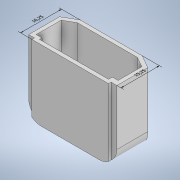
# Autodesk Inventor part: Sarten
Saved by Autodesk Inventor 2020.3 (Build 243373000, 373)
## iProperties
Created: 2021-01-09
Part Number: Sarten
Material: Generic
Document SubType Name: Modeling
Designer: super
Density: 1 g/cm^3
Appearance: Default
Author: super
Autodesk Inventor part; units mm, degrees
ref_plane "YZ Plane" through (0, 0, 0) normal (1, 0, 0) x (0, 1, 0)
ref_plane "XZ Plane" through (0, 0, 0) normal (0, 1, 0) x (-1, 0, 0)
ref_plane "XY Plane" through (0, 0, 0) normal (0, 0, 1) x (1, 0, 0)
sketch "Sketch1" plane through (0, 0, 0) normal (0, 1, 0) x (-1, 0, 0)
  line L0 (0, 0) -> (-35, 0)
  line L1 (-35, 0) -> (-35, -35)
  line L2 (-35, -35) -> (0, -35)
  line L3 (0, -35) -> (0, 0)
  dimension "d0" = 35
  dimension "d1" = 35
  constraints: 8 end point, 2 parallel, 1 horizontal, 1 perpendicular
  measures "d0" distance of L2.end L1.end
  measures "d1" distance of L1.end L0.end
extrude "Extrusion1" add sketch "Sketch1" along normal blind 28
sketch "Sketch2" plane through (0, 28, 0) normal (0, 1, 0) x (1, 0, 0)
  line L0 (35, 19) -> (32.7, 19)
  line L1 (32.7, 19) -> (32.7, 17)
  line L2 (35, 19) -> (35, 17.125)
  line L3 (32.7, 17) -> (35, 17)
  line L4 (35, 17) -> (35, 17.125)
  point P0 (0, 0)
  point P1 (35, 35)
  dimension "d6" = 16
  dimension "d7" = 2.3
  dimension "d8" = 2
  constraints: 10 end point, 2 horizontal, 2 perpendicular
  measures "d6" distance of point (35, 35) L0.start
  measures "d7" distance of L0.start L0.end
  measures "d8" distance of L0.end L1.end
extrude "Extrusion2" cut sketch "Sketch2" against normal blind 28
pattern_linear "Rectangular Pattern1" count 2 spacing 32.7 along (-1, 0, 0) of "Extrusion2"
fillet "Fillet1" radius 6 2 edges at (35, 0, -8.5) (35, 0, -27)
fillet "Fillet2" radius 6 1 edges at (0, 0, -27)
sketch "Sketch3" plane through (0, 28, 0) normal (0, 1, 0) x (1, 0, 0)
  line L0 (6, 0) -> (0, 0) projected
  line L1 (0, 0) -> (0, 3)
  line L2 (0, 17) -> (0, 0) projected
  line L3 (0, 0) -> (3, 0)
  line L4 (0, 3) -> (3, 0)
  dimension "d16" = 3
  constraints: 6 end point, 1 midpoint, 1 point on line
  measures "d16" distance of L0.end L1.end
extrude "Extrusion3" cut sketch "Sketch3" against normal blind 28
sketch "Sketch4" plane through (0, 28, 0) normal (0, 1, 0) x (1, 0, 0)
  line L0 (0, 19) -> (0, 35) projected
  line L1 (0, 35) -> (0, 32)
  line L2 (0, 35) -> (6, 35) projected
  line L3 (0, 35) -> (3, 35)
  line L4 (3, 35) -> (0, 32)
  point P0 (0, 0)
  dimension "d19" = 3
  dimension "d20" = 3
  constraints: 6 end point, 1 midpoint, 1 point on line
  measures "d19" distance of L0.end L1.end
  measures "d20" distance of L0.end L3.end
extrude "Extrusion4" cut sketch "Sketch4" against normal blind 28
sketch "Sketch5" plane through (0, 28, 0) normal (0, 1, 0) x (1, 0, 0)
  line L0 (35, 0) -> (35, 17) projected
  line L1 (35, 0) -> (32, 0)
  line L2 (3, 0) -> (35, 0) projected
  line L3 (35, 0) -> (35, 3)
  line L4 (35, 3) -> (32, 0)
  line L5 (29, 35) -> (35, 35) projected
  line L6 (35, 35) -> (35, 32)
  line L7 (35, 19) -> (35, 35) projected
  line L8 (35, 32) -> (32, 35)
  line L9 (32, 35) -> (35, 35)
  point P0 (0, 0)
  dimension "d23" = 3
  dimension "d24" = 3
  dimension "d25" = 3
  constraints: 12 end point, 3 point on line, 2 perpendicular
  measures "d23" distance of L0.start L1.end
  measures "d24" distance of L0.start L3.end
  measures "d25" distance of L5.end L6.end
extrude "Extrusion5" cut sketch "Sketch5" against normal blind 28
sketch "Sketch6" plane through (0, 28, 0) normal (0, 1, 0) x (1, 0, 0)
  line L0 (3, 0) -> (0, 3) projected
  line L1 (2.3, 17) -> (0, 17) projected
  line L2 (2, 15.75) -> (4.3, 15.75)
  line L3 (4.3, 15.75) -> (4.3, 21.75)
  line L4 (4.3, 21.75) -> (2, 21.75)
  line L5 (0, 19) -> (0, 32) projected
  line L6 (2, 21.75) -> (2, 30.75)
  line L7 (0, 3) -> (0, 5)
  line L8 (0, 17) -> (0, 3) projected
  line L9 (2, 5) -> (2, 15.75)
  line L10 (32, 35) -> (3, 35) projected
  line L11 (3, 35) -> (5, 35)
  line L12 (6, 0) -> (3, 0) projected
  line L13 (3, 0) -> (5, 0)
  line L14 (2.827, 3) -> (2, 3.8818)
  line L15 (2, 3.8818) -> (2, 5)
  line L16 (2.827, 3) -> (3.827, 2)
  line L17 (2.827, 3) -> (4.2412, 3) construction
  line L18 (1.743, 34.4232) -> (3.15, 33.0019)
  line L19 (3.15, 33.0019) -> (2, 31.8635)
  line L20 (2, 31.8635) -> (2, 30.75)
  line L21 (3.15, 33.0019) -> (4.0351, 33.5429)
  line L22 (4.0351, 33.5429) -> (30.1293, 33.5429)
  line L23 (35, 32) -> (32, 35) projected
  line L24 (32.0858, 32.8358) -> (31.3787, 33.5429)
  line L25 (31.3787, 33.5429) -> (30.1293, 33.5429)
  line L26 (35, 19) -> (35, 32) projected
  line L27 (33, 26.25) -> (33, 31.9216)
  line L28 (33, 31.9216) -> (32.0858, 32.8358)
  line L29 (33, 26.25) -> (33, 21.75)
  line L30 (35, 19) -> (32.7, 19) projected
  line L31 (33, 21.75) -> (30.7, 21.75)
  line L32 (30.7, 21.75) -> (30.7, 15.75)
  line L33 (30.7, 15.75) -> (33, 15.75)
  line L34 (33, 15.75) -> (33, 7.3052)
  line L35 (32, 0) -> (35, 3) projected
  line L36 (33.85, 1.85) -> (35.85, 1.85) construction
  line L37 (32.4358, 3.2642) -> (33, 3.8284)
  line L38 (33, 3.8284) -> (33, 7.3052)
  line L39 (27.667, 2) -> (31.1716, 2)
  line L40 (31.1716, 2) -> (32.4358, 3.2642)
  line L41 (27.667, 2) -> (3.827, 2)
  point P0 (0, 0)
  dimension "d31" = 2.3
  dimension "d32" = 6
  dimension "d33" = 2.3
  dimension "d34" = 9
  dimension "d35" = 2
  dimension "d36" = 2
  dimension "d37" = 2
  dimension "d42" = 45
  dimension "d43" = 2
  dimension "d48" = 4.5
  dimension "d49" = 2.3
  dimension "d50" = 6
  dimension "d51" = 2.3
  dimension "d52" = 2
  constraints: 64 end point, 6 perpendicular, 6 point on line, 4 horizontal, 3 vertical, 1 collinear, 1 equal length, 1 parallel
  measures "d31" distance of L2.start L2.end
  measures "d32" distance of L2.end L3.end
  measures "d33" distance of L3.end L4.end
  measures "d34" distance of L4.end L6.end
  measures "d35" distance of L0.end L7.end
  measures "d36" distance of L7.end L9.start
  measures "d37" distance of L10.end L11.end
  measures "d42" angle of L16 L17
  measures "d43" distance of L18.start L18.end
  measures "d48" distance of L27.start L29.end
  measures "d49" distance of L29.end L31.end
  measures "d50" distance of L31.end L32.end
  measures "d51" distance of L32.end L33.end
  measures "d52" distance of L36.start L37.start
extrude "Extrusion6" cut sketch "Sketch6" against normal blind 25.8
sketch "Sketch7" plane through (0, 28, 0) normal (0, 1, 0) x (1, 0, 0)
  line L0 (23.4542, 2) -> (23.9542, 2) construction
  line L1 (32.0858, 2.9142) -> (32.5858, 2.9142) construction
  line L2 (35, 32) -> (32, 35) projected
  line L3 (31.3787, 33.5429) -> (33, 31.9216) projected
  line L4 (2, 31.8635) -> (3.15, 33.0019) projected
  line L5 (2.8776, 32.7322) -> (3.3776, 32.7322) construction
  line L6 (32.4393, 2.5607) -> (31.3787, 1.5)
  line L7 (31.3787, 1.5) -> (23.4542, 1.5)
  line L8 (2.7741, 2.5108) -> (3.7848, 1.5)
  line L9 (3.7848, 1.5) -> (23.4542, 1.5)
  line L10 (2.7741, 2.5108) -> (1.5, 3.7848)
  line L11 (1.5, 3.7848) -> (1.5, 16.2498)
  line L12 (1.5, 16.2498) -> (3.8, 16.2498)
  line L13 (3.8, 16.2498) -> (3.8, 21.2498)
  line L14 (4.3, 21.75) -> (2, 21.75) projected
  line L15 (3.8, 21.2498) -> (1.5, 21.2498)
  line L16 (1.5, 21.2498) -> (1.5, 27.2918)
  line L17 (1.5, 27.2918) -> (1.5, 32.0617)
  line L18 (1.5, 32.0617) -> (2.5241, 33.0858)
  line L19 (2.5241, 33.0858) -> (3.4812, 34.0429)
  line L20 (3.4812, 34.0429) -> (18.3245, 34.0429)
  line L21 (18.3245, 34.0429) -> (31.5858, 34.0429)
  line L22 (31.5858, 34.0429) -> (32.5429, 33.0858)
  line L23 (32.4393, 2.5607) -> (33.5, 3.6213)
  line L24 (33.5, 3.6213) -> (33.5, 11.0333)
  line L25 (33.5, 11.0333) -> (33.5, 16.2503)
  line L26 (33.5, 16.2503) -> (31.2, 16.2503)
  line L27 (30.7, 21.75) -> (30.7, 15.75) projected
  line L28 (31.2, 16.2503) -> (31.2, 21.2503)
  line L29 (31.2, 21.2503) -> (33.5, 21.2503)
  line L30 (33.5, 21.2503) -> (33.5, 32.1287)
  line L31 (33.5, 32.1287) -> (32.5429, 33.0858)
  line L32 (4.0351, 33.5429) -> (31.3787, 33.5429) projected
  line L33 (4.0351, 33.5429) -> (31.3787, 33.5429)
  line L34 (33, 31.9216) -> (33, 21.75) projected
  line L35 (31.3787, 33.5429) -> (33, 31.9216)
  line L36 (33, 31.9216) -> (33, 21.75)
  line L37 (33, 21.75) -> (30.7, 21.75) projected
  line L38 (33, 21.75) -> (30.7, 21.75)
  line L39 (30.7, 21.75) -> (30.7, 15.75)
  line L40 (30.7, 15.75) -> (33, 15.75) projected
  line L41 (31.1716, 2) -> (3.827, 2)
  line L42 (3.827, 2) -> (2.827, 3) projected
  line L43 (2, 3.8818) -> (2, 15.75) projected
  line L44 (3.827, 2) -> (2, 3.8818)
  line L45 (2, 3.8818) -> (2, 15.75)
  line L46 (2, 15.75) -> (4.3, 15.75) projected
  line L47 (2, 15.75) -> (4.3, 15.75)
  line L48 (4.3, 15.75) -> (4.3, 21.75) projected
  line L49 (4.3, 15.75) -> (4.3, 21.75)
  line L50 (4.3, 21.75) -> (2, 21.75)
  line L51 (2, 21.75) -> (2, 31.8635) projected
  line L52 (2, 21.75) -> (2, 31.8635)
  line L53 (3.15, 33.0019) -> (4.0351, 33.5429) projected
  line L54 (2, 31.8635) -> (3.15, 33.0019)
  line L55 (33, 3.8284) -> (31.1716, 2) projected
  line L56 (31.1716, 2) -> (33, 3.8284)
  line L57 (33, 3.8284) -> (33, 15.75)
  line L58 (30.7, 15.75) -> (33, 15.75)
  point P0 (0, 0)
  dimension "d65" = 0.5
  dimension "d70" = 12.465
  dimension "d71" = 2.3
  dimension "d72" = 5
  dimension "d73" = 90
  dimension "d74" = 2.3
  dimension "d76" = 2.3
  dimension "d77" = 5
  dimension "d78" = 2.3
  constraints: 86 end point, 11 perpendicular, 8 collinear, 8 point on line, 5 horizontal, 4 vertical
  measures "d65" distance of L5.start L18.end
  measures "d70" distance of L10.end L11.end
  measures "d71" distance of L11.end L12.end
  measures "d72" distance of L12.end L13.end
  measures "d73" angle of L13 L12
  measures "d74" distance of L13.end L15.end
  measures "d76" distance of L25.end L26.end
  measures "d77" distance of L26.end L28.end
  measures "d78" distance of L28.end L29.end
extrude "Extrusion7" cut sketch "Sketch7" against normal blind 25.8
sketch "Sketch8" plane through (0, 28, 0) normal (0, 1, 0) x (1, 0, 0)
  line L0 (32, 35) -> (35, 32) projected
  line L1 (33.2498, 33.7502) -> (34.7498, 33.7502) construction
  line L2 (29, 35) -> (32, 35) projected
  line L3 (28.3787, 33.5) -> (31.3787, 33.5)
  line L4 (31.3787, 33.5) -> (32.1892, 32.6895)
  line L5 (33.5, 32.1287) -> (33.5, 21.2503) projected
  line L6 (33.5, 31.3787) -> (32.1892, 32.6895)
  line L7 (33.5, 31.3787) -> (33.5, 32.1287)
  line L8 (31.5858, 34.0429) -> (33.5, 32.1287) projected
  line L9 (33.5, 32.1287) -> (31.5858, 34.0429)
  line L10 (3.4812, 34.0429) -> (31.5858, 34.0429) projected
  line L11 (31.5858, 34.0429) -> (3.4812, 34.0429)
  line L12 (1.5, 32.0617) -> (3.4812, 34.0429) projected
  line L13 (3.4812, 34.0429) -> (1.5, 32.0617)
  line L14 (3, 35) -> (0, 32) projected
  line L15 (1.7099, 33.7099) -> (3.2099, 33.7099) construction
  line L16 (2.7705, 32.6492) -> (1.5, 31.3787)
  line L17 (1.5, 21.2498) -> (1.5, 32.0617) projected
  line L18 (4.3449, 35) -> (5.8449, 35) construction
  line L19 (4.3449, 33.5) -> (3.6213, 33.5)
  line L20 (3.6213, 33.5) -> (2.7705, 32.6492)
  line L21 (1.5, 31.3787) -> (1.5, 32.0617)
  line L22 (4.3449, 33.5) -> (28.3787, 33.5)
  point P0 (0, 0)
  dimension "d83" = 1.5
  dimension "d87" = 1.5
  dimension "d89" = 1.5
  constraints: 30 end point, 6 collinear, 6 point on line, 4 horizontal
  measures "d83" distance of L1.start L4.end
  measures "d87" distance of L15.start L16.start
  measures "d89" distance of L18.start L19.start
extrude "Extrusion8" add sketch "Sketch8" against normal blind 25.8
sketch "Sketch9" plane through (0, 28, 0) normal (0, 1, 0) x (1, 0, 0)
  line L0 (0, 3) -> (3, 0) projected
  line L1 (0, 3) -> (5.1962, 0)
  line L2 (3, 0) -> (32, 0) projected
  line L3 (0, 3) -> (6, 3) construction
  line L4 (5.1962, 0) -> (3, 0)
  line L5 (3, 0) -> (0, 3)
  line L6 (35, 17) -> (35, 3) projected
  line L7 (35, 3) -> (29.8038, 0)
  line L8 (32, 0) -> (29, 0) projected
  line L9 (35, 3) -> (41, 3) construction
  line L10 (29.8038, 0) -> (32, 0)
  line L11 (32, 0) -> (35, 3)
  line L12 (35, 19) -> (35, 32) projected
  line L13 (35, 32) -> (29.8038, 35)
  line L14 (29, 35) -> (32, 35) projected
  line L15 (35, 32) -> (41, 32) construction
  line L16 (29.8038, 35) -> (32, 35)
  line L17 (32, 35) -> (35, 32)
  line L18 (0, 19) -> (0, 32) projected
  line L19 (0, 32) -> (5.1962, 35)
  line L20 (3, 35) -> (6, 35) projected
  line L21 (0, 32) -> (6, 32) construction
  line L22 (5.1962, 35) -> (3, 35)
  line L23 (3, 35) -> (0, 32)
  line L24 (0, 32) -> (3, 35) projected
  point P0 (0, 0)
  dimension "d93" = 30
  dimension "d94" = 150
  dimension "d95" = 150
  dimension "d96" = 30
  constraints: 32 end point, 6 point on line, 4 collinear, 4 equal length, 4 horizontal, 2 perpendicular
  measures "d93" angle of L1 L3
  measures "d94" angle of L7 L9
  measures "d95" angle of L15 L13
  measures "d96" angle of L21 L19
extrude "Extrusion9" cut sketch "Sketch9" against normal blind 28
sketch "Sketch10" plane through (0, 28, 0) normal (0, 1, 0) x (1, 0, 0)
  line L0 (1.5, 3.7848) -> (1.5, 16.2498) projected
  line L1 (1.5, 3.7848) -> (5.4575, 1.5)
  line L2 (31.3787, 1.5) -> (3.7848, 1.5) projected
  line L3 (1.5, 3.7848) -> (6.0697, 3.7848) construction
  line L4 (5.4575, 1.5) -> (3.7848, 1.5)
  line L5 (3.7848, 1.5) -> (1.5, 3.7848) projected
  line L6 (3.7848, 1.5) -> (1.5, 3.7848)
  line L7 (33.5, 16.2503) -> (33.5, 3.6213) projected
  line L8 (33.5, 3.6213) -> (29.8258, 1.5)
  line L9 (33.5, 3.6213) -> (37.7426, 3.6213) construction
  line L10 (33.5, 3.6213) -> (31.3787, 1.5) projected
  line L11 (29.8258, 1.5) -> (31.3787, 1.5)
  line L12 (31.3787, 1.5) -> (33.5, 3.6213)
  line L13 (33.5, 31.3787) -> (33.5, 21.2503) projected
  line L14 (33.5, 31.3787) -> (29.8258, 33.5)
  line L15 (3.6213, 33.5) -> (31.3787, 33.5) projected
  line L16 (33.5, 31.3787) -> (37.7426, 31.3787) construction
  line L17 (29.8258, 33.5) -> (31.3787, 33.5)
  line L18 (31.3787, 33.5) -> (33.5, 31.3787)
  line L19 (1.5, 31.3787) -> (3.6213, 33.5) projected
  line L20 (1.5, 31.3787) -> (5.1742, 33.5)
  line L21 (1.5, 31.3787) -> (5.7426, 31.3787) construction
  line L22 (5.1742, 33.5) -> (3.6213, 33.5)
  line L23 (3.6213, 33.5) -> (1.5, 31.3787)
  point P0 (0, 0)
  dimension "d99" = 30
  dimension "d100" = 150
  dimension "d101" = 150
  dimension "d102" = 30
  constraints: 32 end point, 5 horizontal, 5 point on line, 4 collinear, 4 equal length, 1 perpendicular
  measures "d99" angle of L1 L3
  measures "d100" angle of L8 L9
  measures "d101" angle of L16 L14
  measures "d102" angle of L21 L20
extrude "Extrusion10" add sketch "Sketch10" against normal blind 25.8
sketch "Sketch11" plane through (0, 28, 0) normal (0, 1, 0) x (1, 0, 0)
  line L0 (0, 3) -> (5.1962, 0) projected
  line L1 (3.036, 1.2472) -> (4.536, 1.2472) construction
  line L2 (3.786, 2.5462) -> (1.5, 3.866)
  line L3 (1.5, 3.7848) -> (5.4575, 1.5) projected
  line L4 (1.5, 3.866) -> (1.5, 3.7848)
  line L5 (1.5, 3.7848) -> (5.4575, 1.5)
  line L6 (5.4575, 1.5) -> (5.5981, 1.5)
  line L7 (29.8258, 1.5) -> (5.4575, 1.5) projected
  line L8 (5.5981, 1.5) -> (3.786, 2.5462)
  line L9 (29.5815, 1.5) -> (29.8258, 1.5)
  line L10 (33.5, 3.6213) -> (29.8258, 1.5) projected
  line L11 (29.8258, 1.5) -> (33.5, 3.6213)
  line L12 (29.8038, 0) -> (35, 3) projected
  line L13 (32.0253, 1.2826) -> (33.5253, 1.2826) construction
  line L14 (31.2753, 2.5816) -> (33.5, 3.866)
  line L15 (33.5, 16.2503) -> (33.5, 3.6213) projected
  line L16 (33.5, 3.866) -> (33.5, 3.6213)
  line L17 (31.2753, 2.5816) -> (29.4019, 1.5)
  line L18 (29.5815, 1.5) -> (29.4019, 1.5)
  line L19 (29.8038, 35) -> (35, 32) projected
  line L20 (29.8258, 33.5) -> (33.5, 31.3787) projected
  line L21 (32.0253, 33.7174) -> (33.5253, 33.7174) construction
  line L22 (31.2753, 32.4184) -> (29.4019, 33.5)
  line L23 (29.8258, 33.5) -> (5.1742, 33.5) projected
  line L24 (29.8258, 33.5) -> (29.4019, 33.5)
  line L25 (29.8258, 33.5) -> (33.5, 31.3787)
  line L26 (33.5, 31.3787) -> (33.5, 31.134)
  line L27 (33.5, 31.3787) -> (33.5, 21.2503) projected
  line L28 (31.2753, 32.4184) -> (33.5, 31.134)
  line L29 (5.1962, 35) -> (0, 32) projected
  line L30 (2.5981, 33.5) -> (4.0981, 33.5) construction
  line L31 (3.3481, 32.201) -> (1.606, 31.1952)
  line L32 (1.5, 21.2498) -> (1.5, 31.3787) projected
  line L33 (5.1742, 33.5) -> (1.5, 31.3787) projected
  line L34 (1.5, 31.3787) -> (5.1742, 33.5)
  line L35 (5.1742, 33.5) -> (5.5981, 33.5)
  line L36 (3.3481, 32.201) -> (5.5981, 33.5)
  line L37 (1.606, 31.1952) -> (1.5, 31.134)
  line L38 (1.5, 31.3787) -> (1.5, 31.134)
  point P0 (0, 0)
  dimension "d105" = 1.5
  dimension "d109" = 1.5
  dimension "d111" = 1.5
  dimension "d113" = 1.5
  constraints: 52 end point, 12 point on line, 5 horizontal, 5 parallel, 4 collinear, 2 vertical, 1 midpoint, 2 other
  measures "d105" distance of L1.start L2.start
  measures "d109" distance of L13.start L14.start
  measures "d111" distance of L21.start L22.start
  measures "d113" distance of L30.start L31.start
extrude "Extrusion11" add sketch "Sketch11" against normal blind 25.8
sketch "Sketch12" plane through (0, 28, 0) normal (0, 1, 0) x (1, 0, 0)
  line L0 (32.7, 19) -> (32.95, 19) construction
  line L1 (35, 19) -> (35, 32) projected
  line L2 (32.7, 19) -> (32.7, 17) projected
  line L3 (32.7, 19.25) -> (34.2, 19.25) construction
  line L4 (32.7, 20.75) -> (31.2, 20.75)
  line L5 (31.2, 21.2503) -> (31.2, 16.2503) projected
  line L6 (33.5, 21.2503) -> (31.2, 21.2503) projected
  line L7 (31.2, 21.2503) -> (31.2, 20.75)
  line L8 (33.5, 31.134) -> (33.5, 21.2503) projected
  line L9 (31.2, 21.2503) -> (33.5, 21.2503)
  line L10 (33.5, 21.2503) -> (33.5, 20.75)
  line L11 (33.5, 20.75) -> (32.7, 20.75)
  point P0 (0, 0)
  dimension "d117" = 0.25
  dimension "d119" = 1.5
  constraints: 14 end point, 4 perpendicular, 2 horizontal, 2 point on line
  measures "d117" distance of L0.start L3.start
  measures "d119" distance of L3.start L4.start
extrude "Extrusion12" cut sketch "Sketch12" against normal blind 25.8
sketch "Sketch13" plane through (0, 28, 0) normal (0, 1, 0) x (1, 0, 0)
  line L0 (32.7, 19) -> (35, 19) projected
  line L1 (32.7, 19) -> (32.7, 19.25)
  line L2 (32.7, 19.25) -> (35, 19.25)
  line L3 (35, 19.25) -> (35, 19)
  line L4 (32.7, 17) -> (32.7, 19) projected
  line L5 (35, 19) -> (32.7, 19)
  point P0 (0, 0)
  dimension "d123" = 0.25
  constraints: 8 end point, 3 perpendicular, 1 vertical
  measures "d123" distance of L0.start L1.end
extrude "Extrusion13" cut sketch "Sketch13" against normal blind 28
sketch "Sketch14" plane through (0, 28, 0) normal (0, 1, 0) x (1, 0, 0)
  line L0 (32.7, 19.25) -> (35, 19.25) projected
  line L1 (32.7, 19.25) -> (32.7, 19.75)
  line L2 (32.7, 19.75) -> (35, 19.75)
  line L3 (35, 19.25) -> (35, 32) projected
  line L4 (35, 19.75) -> (35, 19.25)
  line L5 (32.7, 17) -> (32.7, 19.25) projected
  line L6 (35, 19.25) -> (32.7, 19.25)
  line L7 (0, 19) -> (2.3, 19) projected
  line L8 (0, 19) -> (0, 19.75)
  line L9 (0, 32) -> (0, 19) projected
  line L10 (0, 19.75) -> (2.3, 19.75)
  line L11 (2.3, 19) -> (2.3, 17) projected
  line L12 (2.3, 19.75) -> (2.3, 19)
  line L13 (2.3, 19) -> (0, 19)
  point P0 (0, 0)
  dimension "d129" = 0.5
  dimension "d130" = 0.75
  constraints: 16 end point, 5 perpendicular, 1 collinear, 1 point on line, 1 vertical
  measures "d129" distance of L0.start L1.end
  measures "d130" distance of L7.start L8.end
extrude "Extrusion14" cut sketch "Sketch14" against normal blind 28
sketch "Sketch15" plane through (0, 28, 0) normal (0, 1, 0) x (1, 0, 0)
  line L0 (0, 19.75) -> (2.3, 19.75) projected
  line L1 (1.15, 17.75) -> (0, 17.75)
  line L2 (0, 17) -> (2.3, 17) projected
  line L3 (0, 17.75) -> (0, 17)
  line L4 (0, 17) -> (2.3, 17)
  line L5 (2.3, 19.75) -> (2.3, 17) projected
  line L6 (1.15, 17.75) -> (2.3, 17.75)
  line L7 (33.2558, 17.75) -> (32.7, 17.75)
  line L8 (32.7, 17) -> (35, 17)
  line L9 (35, 17) -> (35, 17.75)
  line L10 (35, 17.75) -> (33.2558, 17.75)
  line L11 (32.7, 17.75) -> (2.3, 17.75)
  line L12 (2.3, 17) -> (32.7, 17)
  point P0 (0, 0)
  constraints: 20 end point, 3 perpendicular, 3 point on line, 2 horizontal, 2 parallel, 1 collinear
extrude "Extrusion15" add sketch "Sketch15" against normal blind 28
fillet "Fillet5" radius 6 2 edges at (35, 0, -17.375) (0, 0, -17.375)
sketch "Sketch16" plane through (0, 28, 0) normal (0, 1, 0) x (1, 0, 0)
  line L0 (3.8, 16.2498) -> (3.8, 17) projected
  line L1 (31.2, 17.75) -> (3.8, 17.75) projected
  line L2 (3.8, 17) -> (31.2, 17)
  line L3 (31.2, 17) -> (31.2, 17.75)
  line L4 (31.2, 17.75) -> (3.8, 17.75)
  line L5 (3.8, 17.75) -> (3.8, 17)
  point P0 (0, 0)
  constraints: 8 end point, 2 parallel, 1 horizontal, 1 perpendicular
extrude "Extrusion16" cut sketch "Sketch16" against normal blind 25.8
sketch "Sketch17" plane through (0, 28, 0) normal (0, 1, 0) x (1, 0, 0)
  line L0 (33.5, 20.75) -> (31.2, 20.75) projected
  line L1 (33.5, 31.134) -> (33.5, 20.75) projected
  line L2 (31.2, 20.75) -> (33.5, 20.75)
  line L3 (33.5, 20.75) -> (33.5, 21.75)
  line L4 (33.5, 21.75) -> (31.2, 21.75)
  line L5 (31.2, 21.75) -> (31.2, 20.75)
  point P0 (0, 0)
  dimension "d144" = 1
  constraints: 8 end point, 2 parallel, 1 horizontal, 1 perpendicular, 1 point on line
  measures "d144" distance of L3.end L2.end
extrude "Extrusion17" add sketch "Sketch17" against normal blind 25.8
sketch "Sketch18" plane through (0, 28, 0) normal (0, 1, 0) x (1, 0, 0)
  line L0 (31.2, 21.75) -> (31.2, 16.2503) projected
  line L1 (31.2, 18.25) -> (31.2, 19.25)
  line L2 (3.8, 16.2498) -> (3.8, 21.2498) projected
  line L3 (3.8, 18.25) -> (3.8, 19.25)
  line L4 (3.8, 19.25) -> (31.2, 19.25)
  line L5 (31.2, 18.25) -> (3.8, 18.25)
  point P0 (0, 0)
  point P1 (2.3, 17.75)
  dimension "d148" = 1
  constraints: 8 end point, 3 point on line, 2 perpendicular
  measures "d148" distance of L1.start L1.end
extrude "Extrusion18" add sketch "Sketch18" against normal blind 25.8
sketch "Sketch19" plane through (0, 28, 0) normal (0, 1, 0) x (1, 0, 0)
  line L0 (3.8, 18.25) -> (0, 18.25)
  line L1 (0, 18.25) -> (0, 0)
  line L2 (0, 0) -> (35, 0)
  line L3 (35, 0) -> (35, 18.25)
  line L4 (35, 17.75) -> (35, 3) projected
  line L5 (35, 18.25) -> (3.8, 18.25)
  constraints: 10 end point, 3 perpendicular, 1 collinear, 1 horizontal, 1 point on line
extrude "Extrusion19" cut sketch "Sketch19" against normal blind 28
sketch "Sketch20" plane through (0, 28, 0) normal (0, 1, 0) x (1, 0, 0)
  line L0 (3.8, 19.25) -> (3.8, 21.2498) projected
  line L1 (31.2, 21.75) -> (31.2, 19.25) projected
  line L2 (3.8, 19.25) -> (31.2, 19.25)
  line L3 (31.2, 19.25) -> (31.2, 19.75)
  line L4 (31.2, 19.75) -> (3.8, 19.75)
  line L5 (3.8, 19.75) -> (3.8, 19.25)
  point P0 (0, 0)
  dimension "d153" = 0.5
  constraints: 8 end point, 2 parallel, 1 horizontal, 1 perpendicular, 1 point on line
  measures "d153" distance of L3.end L2.end
extrude "Extrusion20" add sketch "Sketch20" against normal blind 25.8
sketch "Sketch21" plane through (0, 28, 0) normal (0, 1, 0) x (1, 0, 0)
  line L0 (2.3, 18.25) -> (32.7, 18.25) projected
  line L1 (32.7, 19.75) -> (32.7, 18.25) projected
  line L2 (2.3, 18.25) -> (32.7, 18.25)
  line L3 (32.7, 18.25) -> (32.7, 18.75)
  line L4 (32.7, 18.75) -> (2.3, 18.75)
  line L5 (2.3, 18.75) -> (2.3, 18.25)
  point P0 (0, 0)
  dimension "d156" = 0.5
  constraints: 8 end point, 2 parallel, 1 horizontal, 1 perpendicular, 1 point on line
  measures "d156" distance of L3.end L2.end
extrude "Extrusion21" cut sketch "Sketch21" against normal blind 28
sketch "Sketch22" plane through (0, 28, 0) normal (0, 1, 0) x (1, 0, 0)
  line L0 (31.2, 19.75) -> (3.8, 19.75) projected
  line L1 (31.2, 21.75) -> (31.2, 19.75) projected
  line L2 (3.8, 19.75) -> (31.2, 19.75)
  line L3 (31.2, 19.75) -> (31.2, 20.25)
  line L4 (31.2, 20.25) -> (3.8, 20.25)
  line L5 (3.8, 20.25) -> (3.8, 19.75)
  point P0 (0, 0)
  dimension "d159" = 0.5
  constraints: 8 end point, 2 parallel, 1 horizontal, 1 perpendicular, 1 point on line
  measures "d159" distance of L3.end L2.end
extrude "Extrusion22" add sketch "Sketch22" against normal blind 25.8
body "Solid1"
